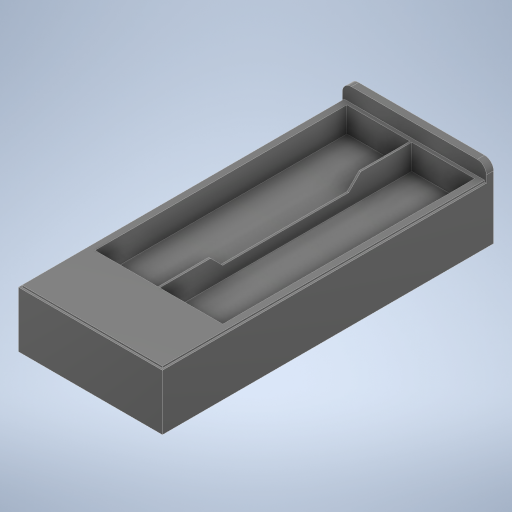
# Autodesk Inventor part: Battery Pack 9.2x4
Saved by Autodesk Inventor 2024 (Build 280153000, 153)
## iProperties
Created: 2023-06-27
Part Number: Battery Pack 9.2x4
Material: PC/ABS Plastic
Document SubType Name: Modeling
Designer: javie
Density: 1.1 g/cm^3
Appearance: Smooth - Black
Author: javie
Autodesk Inventor part; units mm, degrees
ref_plane "YZ Plane" through (0, 0, 0) normal (1, 0, 0) x (0, 1, 0)
ref_plane "XZ Plane" through (0, 0, 0) normal (0, 1, 0) x (-1, 0, 0)
ref_plane "XY Plane" through (0, 0, 0) normal (0, 0, 1) x (1, 0, 0)
sketch "Sketch1" plane through (0, 0, 0) normal (0, 1, 0) x (-1, 0, 0)
  line L0 (-20, 46) -> (20, 46)
  line L1 (20, 46) -> (20, -46)
  line L2 (20, -46) -> (-20, -46)
  line L3 (-20, -46) -> (-20, 46)
  line L4 (-20, 46) -> (20, -46) construction
  line L5 (20, 46) -> (-20, -46) construction
  point P0 (0, 0)
  dimension "d0" = 40
  dimension "d1" = 92
  constraints: 12 end point, 2 midpoint, 2 parallel, 1 horizontal, 1 perpendicular
  measures "d0" distance of L1.end L2.end
  measures "d1" distance of L0.end L1.end
extrude "Extrusion1" add sketch "Sketch1" along normal blind 20
sketch "Sketch2" plane through (0, 20, 0) normal (0, 1, 0) x (1, 0, 0)
  line L0 (-20, 46) -> (-20, -46) projected
  line L1 (20, -46) -> (20, 46) projected
  line L2 (-20, -46) -> (20, -46)
  line L3 (20, -46) -> (20, 44)
  line L4 (20, 44) -> (-20, 44)
  line L5 (-20, 44) -> (-20, -46)
  point P0 (0, 0)
  point P1 (-20, 44)
  dimension "d4" = 90
  constraints: 8 end point, 2 parallel, 1 horizontal, 1 perpendicular, 1 point on line
  measures "d4" distance of L3.end L2.end
extrude "Extrusion2" cut sketch "Sketch2" against normal blind 4
sketch "Sketch3" plane through (0, 16, 0) normal (0, 1, 0) x (1, 0, 0)
  line L0 (0.25, 43) -> (17.75, 43)
  line L1 (17.75, 43) -> (17.75, -27)
  line L2 (17.75, -27) -> (0.25, -27)
  line L3 (0.25, -27) -> (0.25, 43)
  line L4 (20, 44) -> (20, -46) projected
  line L5 (-20, 44) -> (20, 44) projected
  line L6 (-17.75, -27) -> (-0.25, -27)
  line L7 (-0.25, -27) -> (-0.25, 43)
  line L8 (-0.25, 43) -> (-17.75, 43)
  line L9 (-17.75, 43) -> (-17.75, -27)
  line L10 (-20, -46) -> (-20, 44) projected
  point P0 (0, 0)
  dimension "d7" = 17.5
  dimension "d8" = 70
  dimension "d9" = 2.25
  dimension "d10" = 1
  dimension "d11" = 17.5
  dimension "d12" = 2.25
  dimension "d13" = 1
  constraints: 16 end point, 4 parallel, 2 horizontal, 2 perpendicular, 1 point on line
  measures "d7" distance of L1.end L2.end
  measures "d8" distance of L0.end L1.end
  measures "d9" distance between parallel lines of L4 L1
  measures "d10" distance between parallel lines of L5 L0
  measures "d11" distance of L8.end L7.end
  measures "d12" distance between parallel lines of L10 L9
  measures "d13" distance between parallel lines of L5 L8
extrude "Extrusion3" cut sketch "Sketch3" against normal blind 7
sketch "Sketch4" plane through (0.25, 16, 27) normal (1, 0, 0) x (0, 0, -1)
  line L0 (0, 0) -> (70, 0) projected
  line L1 (14.131, 0) -> (17.5, -3.369)
  line L2 (17.5, -3.369) -> (52.5, -3.369)
  line L3 (70, 0) -> (0, 0) projected
  line L4 (52.5, -3.369) -> (55.869, 0)
  line L5 (0, 0) -> (0, -7) projected
  line L6 (70, 0) -> (70, -7) projected
  point P0 (27, -16)
  point P1 (0, -3.5)
  point P2 (70, -3.5)
  dimension "d16" = 45
  dimension "d17" = 45
  dimension "d18" = 17.5
  dimension "d19" = 17.5
  constraints: 6 end point, 2 midpoint, 2 point on line, 1 parallel
  measures "d16" angle of L0 L1
  measures "d17" angle of L0 L4
  measures "d18" horizontal distance of point (0, -3.5) L1.end
  measures "d19" horizontal distance of point (70, -3.5) L2.end
extrude "Extrusion4" cut sketch "Sketch4" against normal up to surface (0.5 mm away)
fillet "Fillet1" radius 2.5 2 edges at (20, 20, -45) (-20, 20, -45)
sketch "Sketch5" plane through (0, 16, 0) normal (0, 1, 0) x (1, 0, 0)
  line L0 (20, 44) -> (20, -46) projected
  line L1 (-20, 44) -> (20, 44)
  line L2 (20, 44) -> (20, -46)
  line L3 (20, -46) -> (-20, -46)
  line L4 (-20, -46) -> (-20, 44)
  line L5 (-19.5, 44.1346) -> (19.5, 44.1346)
  line L6 (19.5, 44.1346) -> (19.5, -45.5)
  line L7 (19.5, -45.5) -> (-19.5, -45.5)
  line L8 (-19.5, -45.5) -> (-19.5, 44.1346)
  line L9 (-17.75, 43) -> (-0.25, 43) projected
  point P0 (0, 0)
  point P1 (19.5, 44)
  point P2 (-19.5, 44)
  dimension "d23" = 0.5
  dimension "d24" = 0.5
  dimension "d25" = 0.5
  constraints: 14 end point, 3 parallel, 2 horizontal, 1 perpendicular, 1 vertical, 3 other
  measures "d23" distance between parallel lines of L4 L8
  measures "d24" distance between parallel lines of L3 L7
  measures "d25" distance between parallel lines of L0 L6
extrude "Extrusion5" cut sketch "Sketch5" against normal blind 0.5 contours L0 L3 L4 L1 L8 L7 L6
body "Solid1"
